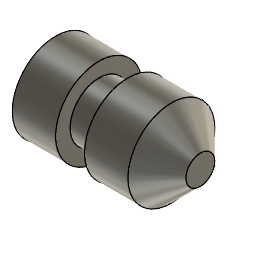
Part2 (Autodesk Fusion 360 design; units mm, degrees)
part number: 2026-06-25-05-23-39-073
Autodesk Fusion 360 part; units mm, degrees
sketch "Sketch1" plane through (0, 0, 0) normal (0, 0, 1) x (1, 0, 0)
  line L0 (0, 0) -> (0, 30)
  line L1 (0, 30) -> (30, 30)
  line L2 (30, 30) -> (30, 20)
  line L3 (30, 20) -> (50, 20)
  line L4 (50, 20) -> (50, 30)
  line L5 (50, 30) -> (80, 30)
  line L6 (80, 30) -> (100, 10)
  line L7 (100, 10) -> (100, 0)
  line L8 (100, 0) -> (0, 0)
  constraint coincident L0.start L8.end
  constraint vertical L0
  constraint perpendicular L0 L1
  constraint perpendicular L1 L2
  constraint perpendicular L2 L3
  constraint perpendicular L1 L4
  constraint perpendicular L4 L5
  constraint perpendicular L5 L7
  constraint perpendicular L0 L8
revolve "Revolve1" add sketch "Sketch1" angle 360 about axis through (100, 0, 0) along (-1, 0, 0)
